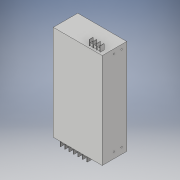
# Autodesk Inventor part: SE600_PS
Saved by Autodesk Inventor 2019 (Build 230136000, 136)
## iProperties
Created: 2019-05-21
Part Number: SE600_PS
Material: Generic
Document SubType Name: Modeling
Designer: Jorian Bruslind
Density: 1 g/cm^3
Appearance: Default
Author: Jorian Bruslind
Autodesk Inventor part; units mm, degrees
ref_plane "YZ Plane" through (0, 0, 0) normal (1, 0, 0) x (0, 1, 0)
ref_plane "XZ Plane" through (0, 0, 0) normal (0, 1, 0) x (-1, 0, 0)
ref_plane "XY Plane" through (0, 0, 0) normal (0, 0, 1) x (1, 0, 0)
sketch "Sketch1" plane through (-63.5, 123.5, 0) normal (0, 0, 1) x (1, 0, 0)
  line L0 (0, 0) -> (127, 0)
  line L1 (127, 0) -> (127, -247)
  line L2 (127, -247) -> (0, -247)
  line L3 (0, -247) -> (0, 0)
  dimension "d0" = 127
  dimension "d1" = 247
  constraints: 8 end point, 2 parallel, 1 horizontal, 1 perpendicular
  measures "d0" distance of L1.end L2.end
  measures "d1" distance of L0.end L1.end
extrude "Extrusion1" add sketch "Sketch1" along normal blind 63.5
sketch "Sketch2" plane through (-63.5, -123.5, 0) normal (0, -1, 0) x (1, 0, 0)
  line L0 (127, 63.5) -> (0, 63.5) projected
  line L1 (0, 63.5) -> (0, 58.5)
  line L2 (0, 0) -> (0, 63.5) projected
  line L3 (0, 58.5) -> (13, 58.5)
  line L4 (13, 58.5) -> (83, 58.5)
  line L5 (83, 58.5) -> (83, 48.5)
  line L6 (83, 48.5) -> (13, 48.5)
  line L7 (13, 48.5) -> (13, 58.5)
  dimension "d8" = 5
  dimension "d7" = 13
  dimension "d5" = 70
  dimension "d6" = 10
  constraints: 12 end point, 2 horizontal, 2 parallel, 1 perpendicular, 1 point on line
  measures "d8" distance of L0.end L1.end
  measures "d7" distance of L1.end L3.end
  measures "d5" distance of L5.end L6.end
  measures "d6" distance of L4.end L5.end
extrude "Extrusion2" add sketch "Sketch2" along normal blind 17
sketch "Sketch3" plane through (63.5, 123.5, 0) normal (0, 1, 0) x (-1, 0, 0)
  line L0 (127, 63.5) -> (0, 63.5) projected
  line L1 (0, 63.5) -> (0, 58.5)
  line L2 (0, 0) -> (0, 63.5) projected
  line L3 (0, 58.5) -> (10, 58.5)
  line L4 (10, 58.5) -> (39.2, 58.5)
  line L5 (39.2, 58.5) -> (39.2, 48.5)
  line L6 (39.2, 48.5) -> (10, 48.5)
  line L7 (10, 48.5) -> (10, 58.5)
  point P0 (127, 0)
  dimension "d15" = 5
  dimension "d14" = 10
  dimension "d12" = 29.2
  dimension "d13" = 10
  constraints: 12 end point, 2 parallel, 2 perpendicular, 1 horizontal, 1 point on line
  measures "d15" distance of L0.end L1.end
  measures "d14" distance of L1.end L3.end
  measures "d12" distance of L5.end L6.end
  measures "d13" distance of L4.end L5.end
extrude "Extrusion3" add sketch "Sketch3" along normal blind 14
sketch "Sketch4" plane through (-63.5, -140.5, 0) normal (0, -1, 0) x (1, 0, 0)
  line L0 (83, 48.5) -> (13, 48.5) projected
  line L1 (13, 58.5) -> (83, 58.5) projected
  line L2 (83, 48.5) -> (81.5, 48.5)
  line L3 (81.5, 48.5) -> (81.5, 58.5)
  line L4 (81.5, 58.5) -> (83, 58.5)
  line L5 (83, 58.5) -> (83, 48.5)
  line L6 (81.5, 48.5) -> (71.5, 48.5)
  line L7 (71.5, 48.5) -> (71.5, 58.5)
  line L8 (71.5, 58.5) -> (81.5, 58.5)
  line L9 (81.5, 58.5) -> (81.5, 48.5)
  point P0 (0, 0)
  dimension "d21" = 1.5
  dimension "d19" = 10
  dimension "d20" = 10
  constraints: 16 end point, 4 parallel, 2 horizontal, 2 perpendicular, 1 point on line
  measures "d21" distance of L3.end L4.end
  measures "d19" distance of L7.end L8.end
  measures "d20" distance of L6.end L7.end
extrude "Extrusion4" cut sketch "Sketch4" against normal blind 8.5 contours L0 L7 L1 L3
sketch "Sketch5" plane through (-63.5, -132, 0) normal (0, -1, 0) x (1, 0, 0)
  circle A0 centre (76.5, 53.5) radius 2.5
  line L0 (81.5, 48.5) -> (71.5, 48.5) projected
  line L1 (71.5, 48.5) -> (71.5, 58.5) projected
  line L2 (81.5, 48.5) -> (83, 48.5) projected
  line L3 (81.5, 48.5) -> (71.5, 48.5)
  line L4 (71.5, 48.5) -> (71.5, 50.25)
  line L5 (71.5, 50.25) -> (81.5, 50.25)
  line L6 (81.5, 50.25) -> (81.5, 48.5)
  line L7 (81.5, 58.5) -> (81.5, 48.5) projected
  line L8 (81.5, 58.5) -> (71.5, 58.5)
  line L9 (71.5, 58.5) -> (71.5, 56.75)
  line L10 (71.5, 56.75) -> (81.5, 56.75)
  line L11 (81.5, 56.75) -> (81.5, 58.5)
  point P0 (0, 0)
  dimension "d29" = 5
  dimension "d31" = 5
  dimension "d30" = 5
  dimension "d27" = 10
  dimension "d28" = 1.75
  dimension "d25" = 10
  dimension "d26" = 1.75
  constraints: 16 end point, 4 parallel, 2 horizontal, 2 perpendicular, 1 centre point
  measures "d29" diameter of A0
  measures "d31" distance from line of L0 A0.centre
  measures "d30" distance from line of L1 A0.centre
  measures "d27" distance of L4.end L5.end
  measures "d28" distance of L3.end L4.end
  measures "d25" distance of L10.end L9.end
  measures "d26" distance of L9.end L8.end
extrude "Extrusion5" cut sketch "Sketch5" against normal blind 8.5 contours A0 | L0 L1 L5 L6 | L10 L1 L8 L7
pattern_linear "Rectangular Pattern1" count 6 spacing 11.5 along (-1, 0, 0) of "Extrusion5", "Extrusion4"
sketch "Sketch6" plane through (63.5, 137.5, 0) normal (0, 1, 0) x (1, 0, 0)
  line L0 (-10, -48.5) -> (-10, -58.5) projected
  line L1 (-10, -48.5) -> (-11, -48.5)
  line L2 (-11, -48.5) -> (-11, -58.5)
  line L3 (-11, -58.5) -> (-10, -58.5)
  line L4 (-10, -58.5) -> (-10, -48.5)
  line L5 (-39.2, -48.5) -> (-10, -48.5) projected
  line L6 (-11, -58.5) -> (-19.2, -58.5)
  line L7 (-19.2, -58.5) -> (-19.2, -48.5)
  line L8 (-19.2, -48.5) -> (-11, -48.5)
  line L9 (-11, -48.5) -> (-11, -58.5)
  point P0 (-63.5, 0)
  dimension "d39" = 1
  dimension "d40" = 8.2
  constraints: 16 end point, 4 parallel, 2 horizontal, 2 perpendicular, 1 point on line
  measures "d39" distance of L3.end L2.end
  measures "d40" distance of L7.end L8.end
extrude "Extrusion6" cut sketch "Sketch6" against normal blind 7 contours L2 L6 L7 L5
sketch "Sketch7" plane through (63.5, 130.5, 0) normal (0, 1, 0) x (1, 0, 0)
  circle A0 centre (-15.1, -53.5) radius 2.5
  line L0 (-19.2, -48.5) -> (-11, -48.5) projected
  line L1 (-11, -48.5) -> (-11, -58.5) projected
  line L2 (-19.2, -58.5) -> (-19.2, -48.5) projected
  line L3 (-19.2, -48.5) -> (-11, -48.5)
  line L4 (-11, -48.5) -> (-11, -50.25)
  line L5 (-11, -50.25) -> (-19.2, -50.25)
  line L6 (-19.2, -50.25) -> (-19.2, -48.5)
  line L7 (-11, -58.5) -> (-19.2, -58.5)
  line L8 (-19.2, -58.5) -> (-19.2, -56.75)
  line L9 (-19.2, -56.75) -> (-11, -56.75)
  line L10 (-11, -56.75) -> (-11, -58.5)
  point P0 (-63.5, 0)
  dimension "d43" = 5
  dimension "d44" = 5
  dimension "d45" = 4.1
  dimension "d46" = 8.2
  dimension "d47" = 1.75
  dimension "d48" = 8.2
  dimension "d49" = 1.75
  constraints: 16 end point, 4 parallel, 2 horizontal, 2 perpendicular, 1 centre point
  measures "d43" diameter of A0
  measures "d44" distance from line of L0 A0.centre
  measures "d45" distance from line of L1 A0.centre
  measures "d46" distance of L4.end L5.end
  measures "d47" distance of L3.end L4.end
  measures "d48" distance of L8.end L9.end
  measures "d49" distance of L7.end L8.end
extrude "Extrusion7" cut sketch "Sketch7" against normal blind 7 contours A0 | L0 L1 L5 L2 | L9 L1 L7 L2
pattern_linear "Rectangular Pattern2" count 3 spacing 9.5 along (-1, 0, 0) of "Extrusion6", "Extrusion7"
sketch "Sketch8" plane through (63.5, -123.5, 0) normal (1, 0, 0) x (0, 0, -1)
  line L0 (-63.5, 247) -> (-63.5, 0) projected
  line L1 (-63.5, 247) -> (-63.5, 236)
  line L2 (-63.5, 236) -> (-13.5, 236)
  circle A0 centre (-13.5, 236) radius 1.75
  point P0 (0, 123.5)
  dimension "d55" = 11
  dimension "d56" = 50
  dimension "d57" = 3.5
  constraints: 4 end point, 1 centre point, 1 coincident, 1 perpendicular, 1 point on line
  measures "d55" distance of L0.start L1.end
  measures "d56" distance of L1.end L2.end
  measures "d57" diameter of A0
extrude "Extrusion8" cut sketch "Sketch8" against normal blind 4
pattern_linear "Rectangular Pattern3" count 2 spacing 220 along (0, -1, 0) count 2 spacing 20 along (0, 0, 1) of "Extrusion8"
mirror "Mirror1" about plane through (0, 0, 0) normal (1, 0, 0) of "Extrusion8", "Rectangular Pattern3"
body "Solid1"
